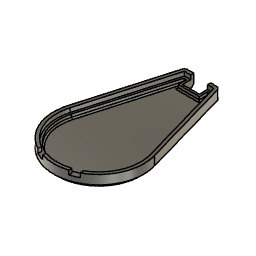
GIXFlashLight (Autodesk Fusion 360 design; units mm, degrees)
Autodesk Fusion 360 part; units mm, degrees
sketch "Sketch1" plane through (0, 0, 0) normal (0, 0, 1) x (1, 0, 0)
  circle A0 centre (0, 0) radius 10
  line L0 (-3, 29.259) -> (3, 29.259)
  line L1 (3, 29.259) -> (3, 23.259)
  line L2 (3, 23.259) -> (-3, 23.259)
  line L3 (-3, 23.259) -> (-3, 29.259)
  line L4 (0, 0) -> (0, 23.259) construction
  line L5 (-3.25, 35.609) -> (3.25, 35.609)
  line L6 (3.25, 35.609) -> (3.25, 42.609)
  line L7 (3.25, 42.609) -> (-3.25, 42.609)
  line L8 (-3.25, 42.609) -> (-3.25, 35.609)
  line L9 (0, 29.259) -> (0, 35.609) construction
  line L10 (-3.25, 38.784) -> (-5.7107, 38.784)
  line L11 (-5.7107, 38.784) -> (-15.577, 4.4802)
  line L12 (0, 0) -> (0, -16.2085) construction
  arc A1 (-15.577, 4.4802) -> (0, -16.2085) centre (0, 0) ccw
  arc A2 (0, -16.2085) -> (15.577, 4.4802) centre (0, 0) ccw
  line L13 (5.7107, 38.784) -> (15.577, 4.4802)
  line L14 (3.25, 38.784) -> (5.7107, 38.784)
  arc A3 (-7.9829, -14.1064) -> (7.9829, -14.1064) centre (0, -16.2085) ccw
  arc A4 (-5.0172, -15.4124) -> (5.0172, -15.4124) centre (0, -16.2085) ccw
  dimension "d1" = 20
  dimension "d2" = 6
  dimension "d3" = 6
  dimension "d4" = 6.5
  dimension "d5" = 7
  dimension "d6" = 16.2085
  dimension "d8" = 15.577
  dimension "d9" = 3.175
  dimension "d10" = 2.4607
  dimension "d11" = 6.35
  dimension "d12" = 5.08
  dimension "d26" = 8.255
  constraint coincident A0.centre L4.start
  constraint horizontal L0
  constraint vertical L1
  constraint horizontal L2
  constraint vertical L3
  constraint midpoint L2 L4.end
  constraint vertical L4
  constraint horizontal L5
  constraint vertical L6
  constraint horizontal L7
  constraint vertical L8
  constraint midpoint L0 L9.start
  constraint midpoint L5 L9.end
  constraint vertical L9
  constraint coincident L8 L10.start
  constraint perpendicular L8 L10
  constraint parallel L4 L12
  constraint tangent L11 A1
  constraint symmetric L9 L10.start L14.start
  constraint symmetric L9 L10.end L13.start
  constraint symmetric L9 L12.end A1.end
  constraint symmetric L9 L11.end A2.end
  constraint symmetric L9 A1 A2
  constraint coincident A1 A3.start
  constraint coincident L12.end A1.end
  constraint coincident A1 A4.start
  constraint coincident A2 A3.end
  constraint coincident A2 A4.end
  measures "d1" diameter of A0
  measures "d2" distance of L0.start L0.end
  measures "d3" distance of L0.start L2.end
  measures "d4" distance of L5.start L5.end
  measures "d5" distance of L5.start L7.end
  measures "d6" radius of A1
  measures "d8" distance of L4 L11.end
  measures "d9" distance of L5 L10
  measures "d10" distance of L10.start L10.end
  measures "d11" distance of L0 L5
  measures "d12" radius of A4
  measures "d26" radius of A3
extrude "Extrude1" add sketch "Sketch1" along normal blind 1.6 contours A0 | L0 L1 L2 L3 | L5 L6 L8 L10 L11 A1 A2 L13 L14 | A1 A2 A3 A4 makes body 1
fillet "Fillet1" [suppressed]
sketch "Sketch3" plane through (0, 0, 1.6) normal (0, 0, 1) x (-1, 0, 0)
  line L0 (-5.7107, -38.784) -> (-3.25, -38.784)
  line L1 (-3.25, -38.784) -> (-3.25, -35.609)
  line L2 (-3.25, -35.609) -> (3.25, -35.609)
  line L3 (3.25, -35.609) -> (3.25, -38.784)
  line L4 (3.25, -38.784) -> (5.7107, -38.784)
  line L5 (5.7107, -38.784) -> (15.577, -4.4802)
  arc A0 (15.577, -4.4802) -> (7.9829, 14.1064) centre (0, 0) ccw
  arc A1 (7.9829, 14.1064) -> (-7.9829, 14.1064) centre (0, 16.2085) ccw
  arc A2 (-7.9829, 14.1064) -> (-15.577, -4.4802) centre (0, 0) ccw
  line L6 (-15.577, -4.4802) -> (-5.7107, -38.784)
  arc A3 (5.0172, 15.4124) -> (0, 16.2085) centre (0, 0) ccw
  arc A4 (5.0172, 15.4124) -> (-5.0172, 15.4124) centre (0, 16.2085) ccw
  line L7 (16.2085, -38.784) -> (-16.2085, -38.784)
  line L8 (-16.2085, -38.784) -> (-16.2085, 24.4635)
  line L9 (-16.2085, 24.4635) -> (16.2085, 24.4635)
  line L10 (16.2085, 24.4635) -> (16.2085, -38.784)
  arc A5 (0, 16.2085) -> (-5.0172, 15.4124) centre (0, 0) ccw
  dimension "d22" = 24.4635
  dimension "d23" = 16.2085
  dimension "d24" = 38.784
  dimension "d25" = 63.2475
  constraint horizontal L7
  constraint vertical L8
  constraint horizontal L9
  constraint vertical L10
  constraint tangent A0 L10
  constraint tangent A2 L8
  constraint tangent A1 L9
  constraint collinear L4 L7
  measures "d22" vertical distance of A0.centre L9.end
  measures "d23" distance of A0.centre L10
  measures "d24" distance of A0.centre L7
  measures "d25" distance of L7 L9
sketch "Sketch6" plane through (0, 0, 1.6) normal (0, 0, 1) x (-1, 0, 0)
  arc A0 (5.0172, 15.4124) -> (0, 16.2085) centre (0, 0) ccw
  arc A1 (0, 16.2085) -> (-5.0172, 15.4124) centre (0, 0) ccw
  arc A2 (5.0172, 15.4124) -> (-5.0172, 15.4124) centre (0, 16.2085) ccw
  line L0 (3.25, -38.784) -> (5.7107, -38.784)
  line L1 (5.7107, -38.784) -> (15.577, -4.4802)
  arc A3 (15.577, -4.4802) -> (7.9829, 14.1064) centre (0, 0) ccw
  arc A4 (7.9829, 14.1064) -> (-7.9829, 14.1064) centre (0, 16.2085) ccw
  arc A5 (-7.9829, 14.1064) -> (-15.577, -4.4802) centre (0, 0) ccw
  line L2 (-15.577, -4.4802) -> (-5.7107, -38.784)
  line L3 (-5.7107, -38.784) -> (-3.25, -38.784)
  line L4 (-3.25, -38.784) -> (-3.25, -35.609)
  line L5 (-3.25, -35.609) -> (3.25, -35.609)
  line L6 (3.25, -35.609) -> (3.25, -38.784)
  line L7 (-2.45, -39.984) -> (-2.45, -36.409)
  line L8 (-2.45, -36.409) -> (2.45, -36.409)
  line L9 (2.45, -36.409) -> (2.45, -39.984)
  line L10 (2.45, -39.984) -> (6.6142, -39.984)
  line L11 (6.6142, -39.984) -> (16.7303, -4.8119)
  arc A6 (9.0375, 14.8788) -> (-9.0375, 14.8788) centre (0, 16.2085) ccw
  arc A7 (-9.0375, 14.8788) -> (-16.7303, -4.8119) centre (0, 0) ccw
  line L12 (-16.7303, -4.8119) -> (-6.6142, -39.984)
  line L13 (-6.6142, -39.984) -> (-2.45, -39.984)
  arc A8 (16.7303, -4.8119) -> (-17.1939, 2.7248) centre (0, 0) ccw
  line L14 (3.25, -38.784) -> (3.25, -39.984)
  line L15 (-3.25, -38.784) -> (-3.25, -39.984)
  arc A9 (-7.0252, 13.7138) -> (-14.8082, -4.2591) centre (0, 0) ccw
  line L16 (-14.8082, -4.2591) -> (-5.1084, -37.984)
  line L17 (-5.1084, -37.984) -> (-4.05, -37.984)
  line L18 (-4.05, -37.984) -> (-4.05, -34.809)
  line L19 (-4.05, -34.809) -> (4.05, -34.809)
  line L20 (4.05, -34.809) -> (4.05, -37.984)
  line L21 (4.05, -37.984) -> (5.1084, -37.984)
  line L22 (5.1084, -37.984) -> (14.8082, -4.2591)
  arc A10 (14.8082, -4.2591) -> (-7.0252, 13.7138) centre (0, 0) ccw
  arc A11 (7.0252, 13.7138) -> (-7.0252, 13.7138) centre (0, 16.2085) ccw
  dimension "d42" = 1.2
  dimension "d43" = 1.2
  dimension "d44" = 1.2
  dimension "d45" = 1.2
  constraint parallel L4 L7
  constraint parallel L5 L8
  constraint parallel L6 L9
  constraint parallel L0 L10
  constraint parallel L1 L11
  constraint concentric A3 A8
  constraint concentric A4 A6
  constraint concentric A5 A7
  constraint parallel L2 L12
  constraint parallel L3 L13
  constraint coincident A6.start A8
  constraint coincident L0.start L6.end
  constraint coincident L10 L14.end
  constraint perpendicular L10 L14
  constraint coincident L3.end L4.start
  constraint perpendicular L3 L15
  constraint concentric A5 A9
  constraint parallel L2 L16
  constraint parallel L3 L17
  constraint parallel L4 L18
  constraint parallel L5 L19
  constraint parallel L6 L20
  constraint parallel L0 L21
  constraint parallel L1 L22
  constraint concentric A3 A10
  constraint concentric A4 A11
  constraint coincident A11.start A10
  constraint coincident A6.end A8
  constraint tangent L11 A8
  constraint tangent A7 L12
  constraint coincident L13 L15.end
  measures "d42" distance of L2 L12
  measures "d43" distance of L1 L11
  measures "d44" distance of L0 L10
  measures "d45" distance of L3 L13
extrude "Extrude2" add sketch "Sketch6" against normal up to surface (1.6 mm away) separate body contours A0 A1 A2 A8 | L0 L1 A3 A4 L10 L11 A8 L14 | A4 A5 L2 L3 A7 L12 L13 A8 L15 makes body 2 at (-4.2356, -16.8854, 1.0667) makes body 3 at (-9.6851, 27.8599, 1.6) makes body 4 at (9.6851, 27.8599, 1.6)
extrude "Extrude3" add sketch "Sketch6" against normal blind 1.5875 from surface at -1.6 contours A0 A1 A2 A8 A10 A11 | A0 A1 A2 A8 | L0 L1 A3 A4 A5 L2 L3 L4 L5 L6 A8 A9 L16 L17 L18 L19 L20 L21 L22 A10 A11 | L0 L1 A3 A4 L10 L11 A8 L14 | A4 A5 L2 L3 A7 L12 L13 A8 L15 bodies 3 4 2
extrude "Extrude4" add sketch "Sketch6" against normal blind 1.5875 from surface at -3.1875 contours A0 A1 A2 A8 A10 A11 | A0 A1 A2 A8 | L0 L1 A3 A4 A5 L2 L3 L4 L5 L6 A8 A9 L16 L17 L18 L19 L20 L21 L22 A10 A11 | L0 L1 A3 A4 L10 L11 A8 L14 | A9 L16 L17 L18 L19 L20 L21 L22 A10 | A4 A5 L2 L3 A7 L12 L13 A8 L15 bodies 3
fillet "Fillet2" radius 1.27 2 edges at (6.6142, 39.984, -0.7875) (-6.6142, 39.984, -0.7875) on bodies 3
chamfer "Chamfer1" distance 1.27 angle 45 3 edges at (11.6722, 22.3979, -3.175) (0, -17.4085, -3.175) (-11.6722, 22.3979, -3.175) on bodies 3
chamfer "Chamfer2" distance 0.508 angle 45 1 faces at (1.35, 14.4424, -1.5875) on bodies 3
sketch "Sketch7" plane through (0, 0, -3.175) normal (0, 0, -1) x (1, 0, 0)
  line L0 (-5.658, -38.714) -> (-3.25, -38.714)
  line L1 (3.25, -38.714) -> (5.658, -38.714)
  line L2 (5.658, -38.714) -> (15.5097, -4.4609)
  arc A0 (15.5097, -4.4608) -> (-15.5097, -4.4608) centre (0, 0) ccw
  line L3 (-15.5097, -4.4608) -> (-5.658, -38.714)
  line L4 (-9.8227, 4.8837) -> (-4.6629, -0.2542)
  line L5 (-4.6629, -0.2542) -> (-8.8607, -4.8455)
  line L6 (-8.8607, -4.8455) -> (-1.8644, -4.8455)
  line L7 (-1.8644, -4.8455) -> (-1.0118, -3.9054)
  line L8 (-1.0118, -3.9054) -> (4.0168, -8.9339)
  line L9 (4.0168, -8.9339) -> (11.2973, -8.9339)
  line L10 (11.2973, -8.9339) -> (2.4426, -0.1449)
  line L11 (2.4426, -0.1449) -> (10.7726, 8.994)
  line L12 (10.7726, 8.994) -> (3.7982, 8.994)
  line L13 (3.7982, 8.994) -> (-1.2304, 3.5063)
  line L14 (-1.2304, 3.5063) -> (-2.6078, 4.8837)
  line L15 (-2.6078, 4.8837) -> (-9.8227, 4.8837)
  line L16 (-3.25, -38.714) -> (-3.25, -35.609)
  line L17 (-3.25, -35.609) -> (3.25, -35.609)
  line L18 (3.25, -35.609) -> (3.25, -38.714)
extrude "Extrude5" cut sketch "Sketch7" against normal blind 0.4 thin wall 0.9906 inside contours L4 L5 L6 L7 L8 L9 L10 L11 L12 L13 L14 L15 bodies 3
hidden bodies 1
equation "d35 = ( -1 / 16 ) * 1 in"
equation "d42 = 0.4 mm * 3"
equation "d43 = 0.4 mm * 3"
equation "d44 = 0.4 mm * 3"
equation "d45 = 0.4 mm * 3"
